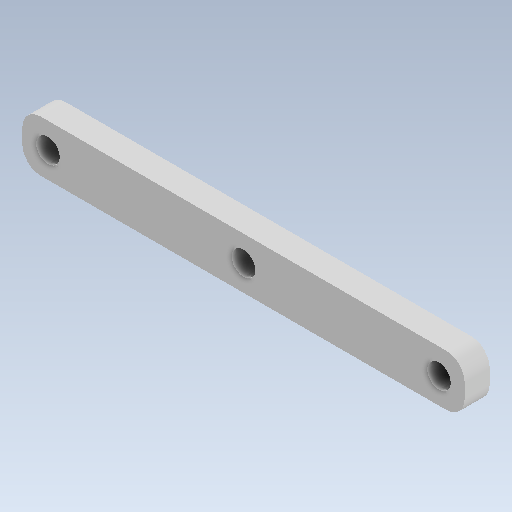
# Autodesk Inventor part: s_arm
Saved by Autodesk Inventor 2020 (Build 240168000, 168)
## iProperties
Created: 2019-10-17
Part Number: s_arm
Material: Generic
Document SubType Name: Modeling
Designer: jesse
Density: 1 g/cm^3
Appearance: Default
Author: jesse
Autodesk Inventor part; units mm, degrees
ref_plane "YZ Plane" through (0, 0, 0) normal (1, 0, 0) x (0, 1, 0)
ref_plane "XZ Plane" through (0, 0, 0) normal (0, 1, 0) x (-1, 0, 0)
ref_plane "XY Plane" through (0, 0, 0) normal (0, 0, 1) x (1, 0, 0)
sketch "Sketch1" plane through (0, 0, 0) normal (0, 0, 1) x (1, 0, 0)
  line L0 (0, 0) -> (56.0985, 0)
  line L1 (56.0985, 0) -> (56.0985, 6.5)
  line L2 (56.0985, 6.5) -> (0, 6.5)
  line L3 (0, 6.5) -> (0, 0)
  line L4 (28.0493, 6.5) -> (28.0493, 0) construction
  circle A0 centre (28.0493, 3.25) radius 1.5
  line L5 (3.25, 6.5) -> (3.25, 0) construction
  line L6 (52.8485, 6.5) -> (52.8485, 0) construction
  circle A1 centre (3.25, 3.25) radius 1.5
  circle A2 centre (52.8485, 3.25) radius 1.5
  line L7 (3.25, 3.25) -> (0, 3.25) construction
  line L8 (52.8485, 3.25) -> (56.0985, 3.25) construction
  line L9 (54.1985, 3.25) -> (54.1985, 0) construction
  dimension "d4" = 3
  dimension "d6" = 6.5
  dimension "d8" = 49.5986
  constraints: 20 end point, 7 midpoint, 6 point on line, 4 perpendicular, 3 centre point, 2 equal length, 2 equal radius, 2 parallel, 1 horizontal
  measures "d4" diameter of A2
  measures "d6" distance between parallel lines of L0 L2
  measures "d8" distance between parallel lines of L5 L6
extrude "Extrusion1" add sketch "Sketch1" along normal blind 3.175
fillet "Fillet1" radius 2.3495 4 edges at (0, 6.5, 1.5875) (0, 0, 1.5875) (56.0985, 6.5, 1.5875) (56.0985, 0, 1.5875)
equation "\"d4\" = hole_size"
equation "\"arm_length\" = support_length"
equation "\"hole_size\" = 3"
equation "\"support_length\" = 58.42"
body "Solid1"
